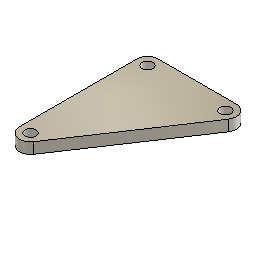
initial (Autodesk Fusion 360 design; units mm, degrees)
Autodesk Fusion 360 part; units mm, degrees
sketch "Sketch1" plane through (0, 0, 0) normal (0, 1, 0) x (1, 0, 0)
  line L0 (0, 6.6056) -> (0, 28)
  line L1 (2, 30) -> (16.263, 30)
  line L2 (17.9271, 26.8906) -> (3.6641, 5.4962)
  arc A0 (2, 30) -> (0, 28) centre (2, 28) ccw
  arc A1 (0, 6.6056) -> (3.6641, 5.4962) centre (2, 6.6056) ccw
  arc A2 (17.9271, 26.8906) -> (16.263, 30) centre (16.263, 28) ccw
  circle A3 centre (2, 28) radius 1
  circle A4 centre (16.263, 28) radius 1
  circle A5 centre (2, 6.6056) radius 1
  point P0 (0, 30)
  point P1 (20, 30)
  dimension "d1" = 20
  dimension "d2" = 30
  dimension "d3" = 2
  dimension "d4" = 2
  dimension "d5" = 2
  dimension "d6" = 2
  dimension "d7" = 2
  dimension "d8" = 2
  constraint vertical L0
  constraint perpendicular L0 L1
  constraint coincident P0 L1
  constraint coincident P0 L0
  constraint tangent L1 A0
  constraint tangent L0 A0
  constraint coincident origin L2
  constraint coincident origin L0
  constraint tangent L2 A1
  constraint tangent L0 A1
  constraint coincident P1 L2
  constraint coincident P1 L1
  constraint tangent L2 A2
  constraint tangent L1 A2
  constraint concentric A0 A3
  constraint concentric A2 A4
  constraint concentric A1 A5
  measures "d1" distance of P0 P1
  measures "d2" distance of origin P0
  measures "d3" radius of A0
  measures "d4" radius of A1
  measures "d5" radius of A2
  measures "d6" diameter of A3
  measures "d7" diameter of A4
  measures "d8" diameter of A5
extrude "Extrude1" add sketch "Sketch1" along normal blind 2
